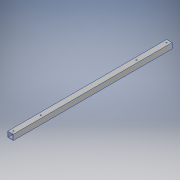
# Autodesk Inventor part: 1by1by6
Saved by Autodesk Inventor 2018 (Build 220112000, 112)
## iProperties
Created: 2018-01-13
Part Number: 1by1by6
Material: Aluminum 6061
Document SubType Name: Modeling
Designer: s-4000369
Density: 2.7 g/cm^3
Appearance: Aluminum - Flat
Mass: 116.143 g
Surface Area: 276.612 cm^2
Volume: 43.016 cm^3
Author: s-4000369
Autodesk Inventor part; units mm, degrees
ref_plane "YZ Plane" through (0, 0, 0) normal (1, 0, 0) x (0, 1, 0)
ref_plane "XZ Plane" through (0, 0, 0) normal (0, 1, 0) x (-1, 0, 0)
ref_plane "XY Plane" through (0, 0, 0) normal (0, 0, 1) x (1, 0, 0)
sketch "Sketch1" plane through (0, 0, 0) normal (1, 0, 0) x (0, 1, 0)
  line L0 (0, 0) -> (25.4, 0)
  line L1 (25.4, 0) -> (25.4, -736.6)
  line L2 (25.4, -736.6) -> (0, -736.6)
  line L3 (0, -736.6) -> (0, 0)
  dimension "d0" = 25.4
  dimension "d1" = 736.6
  constraints: 8 end point, 2 parallel, 1 horizontal, 1 perpendicular
  measures "d0" distance of L0.start L0.end
  measures "d1" distance of L2.end L0.start
extrude "Extrusion1" add sketch "Sketch1" along normal blind 25.4
sketch "Sketch2" plane through (0, 0, 0) normal (0, 0, 1) x (1, 0, 0)
  line L0 (3.175, 3.175) -> (22.225, 3.175)
  line L1 (22.225, 3.175) -> (22.225, 22.225)
  line L2 (22.225, 22.225) -> (3.175, 22.225)
  line L3 (3.175, 22.225) -> (3.175, 3.175)
  line L4 (0, 25.4) -> (25.4, 25.4) projected
  line L5 (0, 0) -> (0, 25.4) projected
  dimension "d4" = 3.175
  dimension "d5" = 3.175
  dimension "d6" = 19.05
  dimension "d7" = 19.05
  constraints: 8 end point, 2 parallel, 1 horizontal, 1 perpendicular
  measures "d4" distance between parallel lines of L2 L4
  measures "d5" distance between parallel lines of L5 L3
  measures "d6" distance of L2.end L0.start
  measures "d7" distance of L0.start L0.end
extrude "Extrusion2" cut sketch "Sketch2" against normal blind 165.1
sketch "Sketch3" plane through (0, 25.4, 0) normal (0, 1, 0) x (1, 0, 0)
  line L0 (0, 0) -> (0, 736.6) projected
  line L1 (0, 0) -> (12.7, 0)
  line L2 (0, 0) -> (25.4, 0) projected
  line L3 (12.7, 0) -> (12.7, 152.4)
  line L4 (22.225, 152.4) -> (3.175, 152.4) projected
  line L5 (12.7, 152.4) -> (12.7, 139.7)
  line L6 (12.7, 0) -> (12.7, 12.7)
  circle A0 centre (12.7, 12.7) radius 2.54
  circle A1 centre (12.7, 139.7) radius 2.54
  dimension "d10" = 152.4
  dimension "d11" = 12.7
  dimension "d12" = 12.7
  dimension "d13" = 5.08
  constraints: 8 end point, 2 centre point, 2 coincident, 2 midpoint, 2 point on line
  measures "d10" distance of L1.end L3.end
  measures "d11" distance of L3.end L5.end
  measures "d12" distance of L1.end L6.end
  measures "d13" diameter of A0
extrude "Extrusion3" cut sketch "Sketch3" against normal blind 25.4
sketch "Sketch4" plane through (0, 25.4, 0) normal (0, 1, 0) x (1, 0, 0)
  line L0 (0, 736.6) -> (25.4, 736.6) projected
  line L1 (12.7, 736.6) -> (0, 736.6)
  line L2 (12.7, 736.6) -> (12.7, 723.9)
  line L3 (12.7, 723.9) -> (12.7, 571.5)
  line L4 (12.7, 571.5) -> (12.7, 584.2)
  circle A0 centre (12.7, 584.2) radius 2.54
  circle A1 centre (12.7, 723.9) radius 2.54
  point P0 (0, 0)
  dimension "d16" = 12.7
  dimension "d17" = 12.7
  dimension "d18" = 152.4
  dimension "d19" = 12.7
  dimension "d20" = 5.08
  constraints: 8 end point, 2 centre point, 2 coincident, 2 point on line, 1 collinear, 1 midpoint, 1 perpendicular
  measures "d16" distance of L1.start L0.start
  measures "d17" distance of L1.start L2.end
  measures "d18" distance of L2.end L3.end
  measures "d19" distance of L3.end L4.end
  measures "d20" diameter of A0
extrude "Extrusion4" cut sketch "Sketch4" against normal blind 25.4
body "Solid1"
